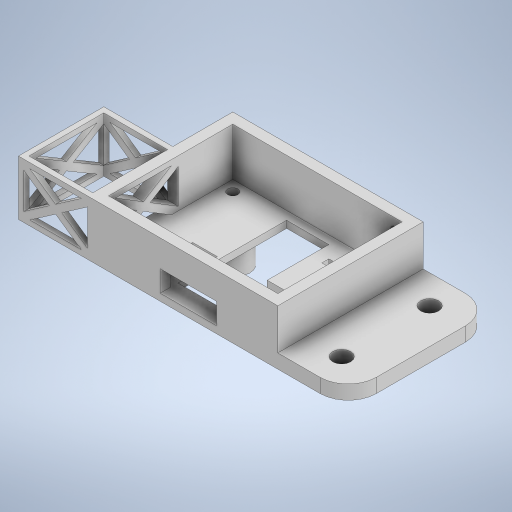
# Autodesk Inventor part: Thermostat_mount
Saved by Autodesk Inventor 2024 (Build 280153000, 153)
## iProperties
Created: 2024-10-23
Part Number: Thermostat_mount
Material: Generic
Document SubType Name: Modeling
Designer: Owner
Density: 1 g/cm^3
Appearance: Default
Author: Owner
Autodesk Inventor part; units mm, degrees
ref_plane "YZ Plane" through (0, 0, 0) normal (1, 0, 0) x (0, 1, 0)
ref_plane "XZ Plane" through (0, 0, 0) normal (0, 1, 0) x (-1, 0, 0)
ref_plane "XY Plane" through (0, 0, 0) normal (0, 0, 1) x (1, 0, 0)
sketch "Sketch1" plane through (0, 0, 0) normal (0, 1, 0) x (-1, 0, 0)
  line L0 (-30.0355, 21.9075) -> (30.0355, 21.9075)
  line L1 (30.0355, 21.9075) -> (30.0355, -21.9075)
  line L2 (30.0355, -21.9075) -> (-30.0355, -21.9075)
  line L3 (-30.0355, -21.9075) -> (-30.0355, 21.9075)
  line L4 (-30.0355, 21.9075) -> (30.0355, -21.9075) construction
  line L5 (30.0355, 21.9075) -> (-30.0355, -21.9075) construction
  line L6 (-30.5435, -22.4155) -> (30.5435, -22.4155)
  line L7 (30.5435, -22.4155) -> (30.5435, 22.4155)
  line L8 (30.5435, 22.4155) -> (-30.5435, 22.4155)
  line L9 (-30.5435, 22.4155) -> (-30.5435, -22.4155)
  line L10 (-28.3845, -20.2565) -> (28.3845, -20.2565)
  line L11 (28.3845, -20.2565) -> (28.3845, 20.2565)
  line L12 (28.3845, 20.2565) -> (-28.3845, 20.2565)
  line L13 (-28.3845, 20.2565) -> (-28.3845, -20.2565)
  line L14 (28.3845, -20.2565) -> (24.9555, -20.2565)
  line L15 (24.9555, -20.2565) -> (24.9555, -16.8275)
  line L16 (24.9555, -16.8275) -> (28.3845, -16.8275)
  line L17 (28.3845, -16.8275) -> (28.3845, -20.2565)
  line L18 (-28.3845, -20.2565) -> (-24.9555, -20.2565)
  line L19 (-24.9555, -20.2565) -> (-24.9555, -16.8275)
  line L20 (-24.9555, -16.8275) -> (-28.3845, -16.8275)
  line L21 (-28.3845, -16.8275) -> (-28.3845, -20.2565)
  line L22 (28.3845, 20.2565) -> (24.9555, 20.2565)
  line L23 (24.9555, 20.2565) -> (24.9555, 16.8275)
  line L24 (24.9555, 16.8275) -> (28.3845, 16.8275)
  line L25 (28.3845, 16.8275) -> (28.3845, 20.2565)
  line L26 (-28.3845, 20.2565) -> (-24.9555, 20.2565)
  line L27 (-24.9555, 20.2565) -> (-24.9555, 16.8275)
  line L28 (-24.9555, 16.8275) -> (-28.3845, 16.8275)
  line L29 (-28.3845, 16.8275) -> (-28.3845, 20.2565)
  circle A0 centre (26.67, -18.542) radius 1.7145
  circle A1 centre (-26.67, -18.542) radius 1.7145
  circle A2 centre (-26.67, 18.542) radius 1.7145
  circle A3 centre (26.67, 18.542) radius 1.7145
  circle A4 centre (26.67, -18.542) radius 1.8415
  circle A5 centre (-26.67, -18.542) radius 1.8415
  circle A6 centre (-26.67, 18.542) radius 1.8415
  circle A7 centre (26.67, 18.542) radius 1.8415
  line L30 (-28.3845, -20.2565) -> (-28.3845, -10.0965)
  line L31 (-30.0355, -21.9075) -> (-30.0355, -11.7475)
  line L32 (-30.0355, -11.7475) -> (-27.4955, -11.7475)
  line L33 (-27.4955, -11.7475) -> (-21.3995, -11.7475)
  line L34 (-21.3995, -11.7475) -> (-21.3995, -4.1275)
  line L35 (-21.3995, -4.1275) -> (-27.4955, -4.1275)
  line L36 (-27.4955, -4.1275) -> (-27.4955, -11.7475)
  line L37 (-30.0355, -21.9075) -> (-14.1605, -21.9075)
  line L38 (-14.1605, -21.9075) -> (-14.1605, -13.6525)
  line L39 (-16.7005, -14.9225) -> (-11.6205, -14.9225)
  line L40 (-11.6205, -14.9225) -> (-11.6205, -12.3825)
  line L41 (-11.6205, -12.3825) -> (-16.7005, -12.3825)
  line L42 (-16.7005, -12.3825) -> (-16.7005, -14.9225)
  line L43 (-16.7005, -14.9225) -> (-11.6205, -12.3825) construction
  line L44 (-11.6205, -14.9225) -> (-16.7005, -12.3825) construction
  line L45 (-30.0355, -21.9075) -> (-7.1755, -21.9075)
  line L46 (-7.1755, -21.9075) -> (-7.1755, -19.3675)
  line L47 (-7.1755, -19.3675) -> (8.0645, -19.3675)
  line L48 (8.0645, -19.3675) -> (8.0645, 2.2225)
  line L49 (8.0645, 2.2225) -> (-7.1755, 2.2225)
  line L50 (-7.1755, 2.2225) -> (-7.1755, -19.3675)
  line L51 (-30.0355, 21.9075) -> (-18.6055, 21.9075)
  line L52 (-18.6055, 21.9075) -> (-18.6055, 13.0175)
  line L53 (-18.6055, 13.0175) -> (8.0645, 13.0175)
  line L54 (8.0645, 13.0175) -> (8.0645, 2.8575)
  line L55 (8.0645, 2.8575) -> (-18.6055, 2.8575)
  line L56 (-18.6055, 2.8575) -> (-18.6055, 13.0175)
  line L57 (-30.0355, 21.9075) -> (-12.2555, 21.9075)
  line L58 (-12.2555, 21.9075) -> (-12.2555, 19.8755)
  line L59 (-12.2555, 19.8755) -> (8.0645, 19.8755)
  line L60 (8.0645, 19.8755) -> (8.0645, 16.0655)
  line L61 (8.0645, 16.0655) -> (-12.2555, 16.0655)
  line L62 (-12.2555, 16.0655) -> (-12.2555, 19.8755)
  line L63 (30.0355, 21.9075) -> (23.0505, 21.9075)
  line L64 (23.0505, 21.9075) -> (19.2405, 21.9075)
  line L65 (19.2405, 21.9075) -> (19.2405, 7.6835)
  line L66 (19.2405, 7.6835) -> (23.0505, 7.6835)
  line L67 (23.0505, 7.6835) -> (23.0505, 21.9075)
  line L68 (30.0355, 21.9075) -> (18.0975, 21.9075)
  line L69 (18.0975, 21.9075) -> (18.0975, 10.4775)
  line L70 (18.0975, 10.4775) -> (9.2075, 10.4775)
  line L71 (9.2075, 10.4775) -> (9.2075, 4.5085)
  line L72 (9.2075, 4.5085) -> (18.0975, 4.5085)
  line L73 (18.0975, 4.5085) -> (18.0975, 10.4775)
  point P0 (0, 0)
  point P1 (-28.3845, -19.214)
  point P2 (-28.3845, -18.542)
  point P3 (-26.67, -16.8275)
  point P4 (-27.342, -16.8275)
  point P5 (23.0505, 20.2565)
  point P6 (19.2405, 20.2565)
  dimension "d0" = 60.071
  dimension "d1" = 43.815
  dimension "d2" = 0.508
  dimension "d3" = 1.651
  dimension "d4" = 3.429
  dimension "d5" = 3.429
  dimension "d6" = 3.429
  dimension "d7" = 3.429
  dimension "d8" = 3.429
  dimension "d9" = 3.683
  dimension "d10" = 3.683
  dimension "d11" = 3.683
  dimension "d12" = 3.683
  dimension "d18" = 10.16
  dimension "d19" = 10.16
  dimension "d20" = 2.54
  dimension "d21" = 6.096
  dimension "d22" = 7.62
  dimension "d23" = 15.875
  dimension "d24" = 8.255
  dimension "d25" = 5.08
  dimension "d26" = 2.54
  dimension "d27" = 22.86
  dimension "d28" = 2.54
  dimension "d29" = 15.24
  dimension "d30" = 21.59
  dimension "d31" = 11.43
  dimension "d32" = 8.89
  dimension "d33" = 26.67
  dimension "d34" = 10.16
  dimension "d35" = 17.78
  dimension "d36" = 2.032
  dimension "d37" = 20.32
  dimension "d38" = 3.81
  dimension "d39" = 6.985
  dimension "d40" = 3.81
  dimension "d41" = 14.224
  dimension "d42" = 11.938
  dimension "d43" = 11.43
  dimension "d44" = 8.89
  dimension "d45" = 5.969
  constraints: 148 end point, 28 parallel, 20 perpendicular, 12 horizontal, 12 tangent, 11 point on line, 8 centre point, 4 coincident, 4 midpoint, 6 other
  measures "d0" distance of L1.end L2.end
  measures "d1" distance of L0.end L1.end
  measures "d2" distance between parallel lines of L2 L6
  measures "d3" distance between parallel lines of L2 L10
  measures "d4" distance of L15.end L16.end
  measures "d5" distance of L14.end L15.end
  measures "d6" distance of L20.end L19.end
  measures "d7" distance of L19.end L18.end
  measures "d8" distance of L23.end L22.end
  measures "d9" diameter of A4
  measures "d10" diameter of A5
  measures "d11" diameter of A6
  measures "d12" diameter of A7
  measures "d18" distance of L10.start L30.end
  measures "d19" distance of L2.end L31.end
  measures "d20" distance of L31.end L32.end
  measures "d21" distance of L35.end L34.end
  measures "d22" distance of L34.end L33.end
  measures "d23" distance of L2.end L37.end
  measures "d24" distance of L37.end L38.end
  measures "d25" distance of L41.end L40.end
  measures "d26" distance of L40.end L39.end
  measures "d27" distance of L2.end L45.end
  measures "d28" distance of L45.end L46.end
  measures "d29" distance of L49.end L48.end
  measures "d30" distance of L48.end L47.end
  measures "d31" distance of L0.start L51.end
  measures "d32" distance of L51.end L52.end
  measures "d33" distance of L54.end L55.end
  measures "d34" distance of L53.end L54.end
  measures "d35" distance of L0.start L57.end
  measures "d36" distance of L57.end L58.end
  measures "d37" distance of L60.end L61.end
  measures "d38" distance of L59.end L60.end
  measures "d39" distance of L0.end L63.end
  measures "d40" distance of L66.end L65.end
  measures "d41" distance of L65.end L64.end
  measures "d42" distance of L0.end L68.end
  measures "d43" distance of L68.end L69.end
  measures "d44" distance of L72.end L71.end
  measures "d45" distance of L71.end L70.end
extrude "Extrusion1" add sketch "Sketch1" along normal blind 2.54 contours L0 L52 L12 A6 L13 L32 L3 | L0 L58 L12 L52 | L32 L13 A5 L10 L38 L2 L3 | L0 L69 L12 L58 | L12 L65 L66 L67 L23 A7 L24 L11 L16 A4 L15 L10 L19 A5 L20 L13 L28 A6 L27 | L0 L65 L12 L69 | L27 A6 L12 | L38 L10 L46 L2 | L20 A5 L13 | L0 L67 L12 L65 | L46 L10 A4 L11 A7 L12 L67 L0 L1 L2 | L13 A6 L28 | A5 L20 A1 L13 | L13 A5 | A6 L13 L12 | L10 A5 L19 | A5 L10 L13 | L20 L19 A5 | L27 L28 A6 | L15 A4 L10 | L12 A7 L23 | A4 L11 L10 | L15 L16 A4 | L12 L11 A7 | A7 L24 L23 | A4 L16 L11 | L11 L24 A7 | L9 L8 L7 L6
sketch "Sketch2" plane through (0, 0, 0) normal (0, -1, 0) x (1, 0, 0)
  line L0 (-30.5435, 22.4155) -> (30.5435, 22.4155) projected
  line L1 (-30.5435, -22.4155) -> (30.5435, -22.4155)
  line L2 (30.5435, -22.4155) -> (30.5435, 22.4155)
  line L3 (30.5435, 22.4155) -> (-30.5435, 22.4155)
  line L4 (-30.5435, 22.4155) -> (-30.5435, -22.4155)
  line L5 (-30.5435, -22.4155) -> (30.5435, 22.4155) construction
  line L6 (30.5435, -22.4155) -> (-30.5435, 22.4155) construction
  line L7 (-34.3535, -26.2255) -> (34.3535, -26.2255)
  line L8 (34.3535, -26.2255) -> (34.3535, 26.2255)
  line L9 (34.3535, 26.2255) -> (-34.3535, 26.2255)
  line L10 (-34.3535, 26.2255) -> (-34.3535, -26.2255)
  line L11 (-30.5435, 22.4155) -> (-34.3535, 22.4155)
  line L12 (-34.3535, 22.4155) -> (34.3535, 22.4155)
  line L13 (-34.3535, -22.4155) -> (34.3535, -22.4155)
  point P0 (0, 0)
  dimension "d15" = 3.81
  constraints: 26 end point, 7 point on line, 4 parallel, 3 perpendicular, 2 midpoint, 1 horizontal, 3 other
  measures "d15" distance between parallel lines of L4 L10
extrude "Extrusion2" add sketch "Sketch2" against normal blind 19.812 contours L11 L10 L9 L8 L12 L0 | L4 L13 L10 L11 | L12 L8 L13 L2 | L1 L13 L8 L7 L10
sketch "Sketch3" plane through (-34.3535, 0, 26.2255) normal (0, 0, 1) x (1, 0, 0)
  line L0 (3.81, 2.54) -> (64.897, 2.54) projected
  line L1 (64.897, 2.54) -> (68.707, 2.54)
  line L2 (68.707, 0) -> (68.707, 19.812) projected
  line L3 (64.897, 2.54) -> (64.897, 0)
  line L4 (68.707, 2.54) -> (46.609, 2.54)
  line L5 (46.609, 2.54) -> (26.289, 2.54)
  line L6 (26.289, 2.54) -> (26.289, 10.16)
  line L7 (26.289, 10.16) -> (46.609, 10.16)
  line L8 (46.609, 10.16) -> (46.609, 2.54)
  point P0 (34.3535, 0)
  point P1 (26.289, 2.54)
  dimension "d46" = 22.098
  dimension "d47" = 20.32
  dimension "d48" = 7.62
  constraints: 14 end point, 2 horizontal, 2 parallel, 2 point on line, 1 perpendicular, 1 vertical
  measures "d46" distance of L1.end L4.end
  measures "d47" distance of L6.end L7.end
  measures "d48" distance of L5.end L6.end
extrude "Extrusion3" cut sketch "Sketch3" against normal blind 3.81
sketch "Sketch4" plane through (34.3535, 0, 26.2255) normal (1, 0, 0) x (0, 0, -1)
  line L0 (52.451, 0) -> (0, 0) projected
  line L1 (0, 10.16) -> (0, 2.54) projected
  line L2 (52.451, 0) -> (0, 0)
  line L3 (0, 0) -> (0, 5.08)
  line L4 (0, 5.08) -> (52.451, 5.08)
  line L5 (52.451, 5.08) -> (52.451, 0)
  point P0 (26.2255, 0)
  dimension "d51" = 5.08
  constraints: 8 end point, 2 parallel, 1 horizontal, 1 perpendicular, 1 point on line
  measures "d51" distance of L2.end L3.end
extrude "Extrusion4" add sketch "Sketch4" along normal blind 25.4
sketch "Sketch5" plane through (34.3535, 5.08, 26.2255) normal (0, 1, 0) x (1, 0, 0)
  line L0 (-68.707, 52.451) -> (25.4, 52.451) projected
  line L1 (0, 0) -> (0, 52.451) projected
  line L2 (25.4, 52.451) -> (0, 52.451)
  line L3 (0, 52.451) -> (0, 0)
  line L4 (0, 0) -> (25.4, 0)
  line L5 (25.4, 0) -> (25.4, 52.451)
  line L6 (12.7, 52.451) -> (12.7, 0)
  line L7 (25.4, 26.2255) -> (0, 26.2255)
  line L8 (0, 10.3505) -> (25.4, 10.3505)
  line L9 (25.4, 10.3505) -> (25.4, 42.1005)
  line L10 (25.4, 42.1005) -> (0, 42.1005)
  line L11 (0, 42.1005) -> (0, 10.3505)
  line L12 (0, 10.3505) -> (25.4, 42.1005) construction
  line L13 (25.4, 10.3505) -> (0, 42.1005) construction
  circle A0 centre (12.7, 42.1005) radius 3.2385
  circle A1 centre (12.7, 10.3505) radius 3.2385
  point P0 (-34.3535, 26.2255)
  point P1 (12.7, 26.2255)
  dimension "d54" = 25.4
  dimension "d55" = 31.75
  dimension "d56" = 6.477
  dimension "d57" = 6.477
  constraints: 24 end point, 9 midpoint, 4 parallel, 2 centre point, 2 horizontal, 2 perpendicular
  measures "d54" distance of L10.end L9.end
  measures "d55" distance of L9.end L8.end
  measures "d56" diameter of A0
  measures "d57" diameter of A1
extrude "Extrusion5" cut sketch "Sketch5" against normal blind 25.4 contours A0 L10 L6 | L6 L10 A0 | L10 L6 A0 | L10 A0 L6 | A1 L6 L8 | L8 L6 A1 | A1 L8 L6 | L8 A1 L6
fillet "Fillet1" radius 10.16 2 edges at (59.7535, 2.54, -26.2255) (59.7535, 2.54, 26.2255)
sketch "Sketch6" plane through (0, 0, 0) normal (0, -1, 0) x (1, 0, 0)
  circle A0 centre (-26.67, -18.542) radius 1.8415 projected
  line L0 (-24.8285, -18.542) -> (-5.6313, -18.542)
  line L1 (-5.6313, -18.542) -> (-5.6313, 2.1308)
  line L2 (-5.6313, 2.1308) -> (-24.8285, 2.1308)
  line L3 (-24.8285, 2.1308) -> (-24.8285, -18.542)
  line L4 (-5.6313, -8.2056) -> (-24.8285, -8.2056)
  line L5 (-15.2299, -18.542) -> (-15.2299, 2.1308)
  circle A1 centre (-15.2299, -8.2056) radius 5.08
  point P0 (0, 0)
  dimension "d61" = 10.16
  constraints: 12 end point, 5 midpoint, 2 parallel, 1 centre point, 1 horizontal, 1 horizontal alignment, 1 perpendicular, 1 other
  measures "d61" diameter of A1
extrude "Extrusion6" add sketch "Sketch6" along normal blind 9.398 contours A1 L4 L5 | L5 L4 A1 | A1 L5 L4 | L5 A1 L4
sketch "Sketch7" plane through (0, 0, 0) normal (0, -1, 0) x (1, 0, 0)
  line L0 (-8.0645, 2.2225) -> (-8.0645, -19.3675) projected
  line L1 (-8.0645, 2.2225) -> (-8.0645, 2.8575)
  line L2 (-8.0645, 2.8575) -> (18.6055, 2.8575) projected
  line L3 (7.1755, -19.3675) -> (7.1755, 2.2225) projected
  line L4 (7.1755, 2.2225) -> (-8.0645, 2.2225)
  line L5 (-8.0645, 2.2225) -> (-8.0645, 2.8575)
  line L6 (-8.0645, 2.8575) -> (7.1755, 2.8575)
  line L7 (7.1755, 2.8575) -> (7.1755, 2.2225)
  point P0 (0, 0)
  point P1 (7.1755, 2.8575)
  constraints: 10 end point, 2 parallel, 1 horizontal, 1 perpendicular, 1 point on line, 1 vertical
extrude "Extrusion7" cut sketch "Sketch7" against normal blind 9.398
sketch "Sketch8" plane through (34.3535, 19.812, -26.2255) normal (0, 0, -1) x (-1, 0, 0)
  line L0 (22.098, -17.272) -> (3.81, -17.272) projected
  line L1 (3.81, 0) -> (64.897, 0) projected
  line L2 (3.81, -17.272) -> (3.81, 0)
  line L3 (59.182, -17.272) -> (62.865, -17.272) projected
  line L4 (3.81, -17.272) -> (62.865, -17.272)
  circle A0 centre (5.969, -4.6996) radius 2.159
  point P0 (34.3535, -19.812)
  dimension "d66" = 4.318
  constraints: 4 end point, 1 centre point, 1 horizontal, 1 perpendicular, 1 tangent
  measures "d66" diameter of A0
extrude "Extrusion8" cut sketch "Sketch8" against normal blind 25.4
sketch "Sketch9" plane through (0, 0, 0) normal (0, -1, 0) x (1, 0, 0)
  line L0 (-34.3535, 26.2255) -> (-34.3535, 24.3205)
  line L1 (-34.3535, 26.2255) -> (-34.3535, -26.2255) projected
  line L2 (-34.3535, 24.3205) -> (-57.3535, 24.3205)
  line L3 (-57.3535, 24.3205) -> (-57.3535, -2.6795)
  line L4 (-57.3535, -2.6795) -> (-34.3535, -2.6795)
  line L5 (-34.3535, -2.6795) -> (-34.3535, 24.3205)
  line L6 (-59.2585, -4.5845) -> (-59.2585, 26.2255)
  line L7 (-59.2585, 26.2255) -> (-32.4485, 26.2255)
  line L8 (-32.4485, 26.2255) -> (-32.4485, -4.5845)
  line L9 (-32.4485, -4.5845) -> (-59.2585, -4.5845)
  line L10 (-34.3535, 26.2255) -> (-34.3535, -4.5845)
  point P0 (0, 0)
  dimension "d69" = 1.905
  dimension "d70" = 23
  dimension "d71" = 27
  dimension "d72" = 1.905
  constraints: 20 end point, 4 parallel, 3 point on line, 2 perpendicular, 1 horizontal, 3 other
  measures "d69" distance of L0.start L0.end
  measures "d70" distance of L4.end L3.end
  measures "d71" distance of L3.end L2.end
  measures "d72" distance between parallel lines of L3 L6
extrude "Extrusion9" add sketch "Sketch9" against normal up to surface (19.812 mm away) contours L0 L2 L3 L4 L1 L9 L6 L7
sketch "Sketch10" plane through (-34.3535, 0, -2.6795) normal (-1, 0, 0) x (0, 0, 1)
  line L0 (0, 19.812) -> (27, 19.812) projected
  line L1 (0, 19.812) -> (0, 0) projected
  line L2 (27, 19.812) -> (0, 19.812)
  line L3 (0, 19.812) -> (0, 17.907)
  line L4 (0, 17.907) -> (27, 17.907)
  line L5 (27, 17.907) -> (27, 19.812)
  point P0 (2.6795, 0)
  dimension "d75" = 1.905
  constraints: 8 end point, 2 parallel, 1 horizontal, 1 perpendicular, 1 point on line
  measures "d75" distance of L3.end L2.end
extrude "Extrusion10" add sketch "Sketch10" along normal up to surface (23 mm away)
sketch "Sketch11" plane through (34.3535, 5.08, 26.2255) normal (0, 0, 1) x (1, 0, 0)
  line L0 (-91.707, 12.827) -> (-68.707, 12.827) projected
  line L1 (-91.707, -5.08) -> (-91.707, 12.827) projected
  line L2 (-68.707, 12.827) -> (-91.707, 12.827)
  line L3 (-91.707, 12.827) -> (-91.707, -3.175)
  line L4 (-91.707, -3.175) -> (-68.707, -3.175)
  line L5 (-68.707, -3.175) -> (-68.707, 12.827)
  line L6 (-91.707, 12.827) -> (-68.707, -3.175)
  line L7 (-91.707, -3.175) -> (-68.707, 12.827)
  line L8 (-90.9817, 13.8695) -> (-67.9817, -2.1325)
  line L9 (-92.4323, 11.7845) -> (-69.4323, -4.2175)
  line L10 (-92.4323, -2.1325) -> (-69.4323, 13.8695)
  line L11 (-90.9817, -4.2175) -> (-67.9817, 11.7845)
  point P0 (-34.3535, -5.08)
  point P1 (-80.207, 3.2789)
  point P2 (-89.4833, -3.175)
  point P3 (-70.9307, -3.175)
  point P4 (-68.707, 11.2799)
  point P5 (-77.9833, 4.826)
  point P6 (-68.707, -1.6279)
  point P7 (-91.707, -1.6279)
  point P8 (-82.4307, 4.826)
  point P9 (-91.707, 11.2799)
  point P10 (-80.207, 6.3731)
  point P11 (-70.9307, 12.827)
  point P12 (-89.4833, 12.827)
  dimension "d78" = 16.002
  dimension "d79" = 1.27
  dimension "d80" = 1.27
  dimension "d81" = 1.27
  dimension "d82" = 1.27
  constraints: 20 end point, 6 parallel, 1 horizontal, 1 perpendicular, 1 point on line
  measures "d78" distance of L3.end L2.end
  measures "d79" distance between parallel lines of L6 L8
  measures "d80" distance between parallel lines of L6 L9
  measures "d81" distance between parallel lines of L7 L10
  measures "d82" distance between parallel lines of L7 L11
extrude "Extrusion11" cut sketch "Sketch11" against normal blind 50.8 contours L0 L10 L8 | L9 L10 L1 | L5 L8 L11 | L11 L9 L4
sketch "Sketch12" plane through (-59.2585, 0, -4.5845) normal (-1, 0, 0) x (0, 0, 1)
  line L0 (1.905, 17.907) -> (28.905, 17.907) projected
  line L1 (1.905, 17.907) -> (28.9052, 17.907)
  line L2 (28.9052, 17.907) -> (28.9052, 1.905)
  line L3 (28.9052, 1.905) -> (1.905, 1.905)
  line L4 (1.905, 1.905) -> (1.905, 17.907)
  line L5 (1.905, 17.907) -> (28.9052, 1.905)
  line L6 (1.905, 1.905) -> (28.9052, 17.907)
  line L7 (1.2575, 2.9975) -> (28.2577, 18.9995)
  line L8 (2.5525, 0.8125) -> (29.5527, 16.8145)
  line L9 (2.5525, 18.9995) -> (29.5527, 2.9975)
  line L10 (1.2575, 16.8145) -> (28.2577, 0.8125)
  point P0 (4.5845, 0)
  point P1 (26.4143, 1.905)
  point P2 (15.4051, 8.4297)
  point P3 (4.3959, 1.905)
  point P4 (17.896, 9.906)
  point P5 (28.9052, 3.3813)
  point P6 (28.9052, 16.4307)
  point P7 (12.9142, 9.906)
  point P8 (1.905, 16.4307)
  point P9 (1.905, 3.3813)
  point P10 (4.3959, 17.907)
  point P11 (15.4051, 11.3823)
  point P12 (26.4143, 17.907)
  dimension "d85" = 27.0002
  dimension "d86" = 16.002
  dimension "d87" = 1.27
  dimension "d88" = 1.27
  dimension "d89" = 1.27
  dimension "d90" = 1.27
  constraints: 20 end point, 6 parallel, 1 horizontal, 1 perpendicular
  measures "d85" distance of L2.end L3.end
  measures "d86" distance of L1.end L2.end
  measures "d87" distance between parallel lines of L6 L7
  measures "d88" distance between parallel lines of L6 L8
  measures "d89" distance between parallel lines of L5 L9
  measures "d90" distance between parallel lines of L5 L10
extrude "Extrusion12" cut sketch "Sketch12" against normal blind 2.54 contours L0 L7 L9 | L10 L7 L4 | L2 L9 L8 | L8 L10 L3
sketch "Sketch13" plane through (-30.5435, 2.54, -22.4155) normal (1, 0, 0) x (0, 0, -1)
  line L0 (-44.831, 17.272) -> (-44.831, 15.367)
  line L1 (-19.736, 15.367) -> (-19.736, 13.8199) projected
  line L2 (-44.831, 15.367) -> (-19.736, 15.367)
  line L3 (-19.736, 15.367) -> (-19.736, 0)
  line L4 (0, 0) -> (-44.831, 0) projected
  line L5 (-19.736, 0) -> (-44.831, 0)
  line L6 (-44.831, 0) -> (-44.831, 15.367)
  line L7 (-19.736, 0) -> (-44.831, 15.367)
  line L8 (-44.831, 0) -> (-19.736, 15.367)
  line L9 (-20.3992, -1.0831) -> (-45.4942, 14.2839)
  line L10 (-19.0728, 1.0831) -> (-44.1678, 16.4501)
  line L11 (-45.4942, 1.0831) -> (-20.3992, 16.4501)
  line L12 (-44.1678, -1.0831) -> (-19.0728, 14.2839)
  point P0 (-22.4155, -2.54)
  point P1 (-19.736, 13.8778)
  point P2 (-29.8516, 7.6835)
  point P3 (-19.736, 1.4892)
  point P4 (-32.2835, 9.1727)
  point P5 (-22.1679, 15.367)
  point P6 (-42.3991, 15.367)
  point P7 (-32.2835, 6.1943)
  point P8 (-42.3991, 0)
  point P9 (-22.1679, 0)
  point P10 (-44.831, 1.4892)
  point P11 (-34.7154, 7.6835)
  point P12 (-44.831, 13.8778)
  dimension "d93" = 1.905
  dimension "d94" = 1.27
  dimension "d95" = 1.27
  dimension "d96" = 1.27
  dimension "d97" = 1.27
  constraints: 22 end point, 4 parallel, 2 vertical, 1 collinear, 1 point on line
  measures "d93" distance of L0.start L0.end
  measures "d94" distance between parallel lines of L7 L9
  measures "d95" distance between parallel lines of L7 L10
  measures "d96" distance between parallel lines of L8 L11
  measures "d97" distance between parallel lines of L8 L12
extrude "Extrusion13" cut sketch "Sketch13" against normal blind 5.08 contours L1 L3 L10 L12 | L11 L10 L2 | L9 L4 L12 | L9 L11 L6
sketch "Sketch14" plane through (0, 19.812, 0) normal (0, 1, 0) x (1, 0, 0)
  line L0 (-34.3535, 2.6795) -> (-34.3535, 4.5845) projected
  line L1 (-57.3535, -21.8298) -> (-57.3535, -24.3205) projected
  line L2 (-34.3535, 2.6795) -> (-57.3535, 2.6795)
  line L3 (-57.3535, 2.6795) -> (-57.3535, -24.3205)
  line L4 (-57.3535, -24.3205) -> (-34.3535, -24.3205)
  line L5 (-34.3535, -24.3205) -> (-34.3535, 2.6795)
  line L6 (-57.3535, 2.6795) -> (-34.3535, -24.3205)
  line L7 (-34.3535, -24.3205) -> (-34.3535, 2.6795) projected
  line L8 (-57.3535, -26.2255) -> (-57.3535, -24.3207) projected
  line L9 (-34.3535, 2.6795) -> (-57.3535, -24.3207)
  line L10 (-56.3867, 3.5031) -> (-33.3867, -23.4969)
  line L11 (-58.3203, 1.8559) -> (-35.3203, -25.1441)
  line L12 (-35.3203, 3.503) -> (-58.6235, -23.8531)
  line L13 (-58.6235, -23.8531) -> (-58.6235, -26.2255)
  line L14 (-33.3867, 1.856) -> (-56.0835, -24.7883)
  line L15 (-56.0835, -24.7883) -> (-56.0835, -26.2255)
  line L16 (-50.9335, -16.7841) -> (-40.7735, -16.7841)
  line L17 (-40.7735, -16.7841) -> (-40.7735, -4.8571)
  line L18 (-40.7735, -4.8571) -> (-50.9335, -4.8571)
  line L19 (-50.9335, -4.8571) -> (-50.9335, -16.7841)
  line L20 (-50.9335, -16.7841) -> (-40.7735, -4.8571) construction
  line L21 (-40.7735, -16.7841) -> (-50.9335, -4.8571) construction
  point P0 (0, 0)
  point P1 (-45.8535, -10.8206)
  point P2 (-42.4417, -16.7841)
  point P3 (-49.2652, -16.7841)
  point P4 (-55.685, -24.3205)
  point P5 (-36.0218, -24.3205)
  point P6 (-40.7735, -6.8156)
  point P7 (-40.7735, -14.8255)
  point P8 (-34.3535, -22.362)
  point P9 (-34.3535, 0.721)
  point P10 (-50.9335, -14.8256)
  point P11 (-50.9335, -6.8155)
  point P12 (-57.3535, 0.721)
  point P13 (-57.3535, -22.3622)
  point P14 (-49.2651, -4.8571)
  point P15 (-42.4418, -4.8571)
  point P16 (-36.0218, 2.6795)
  point P17 (-55.6852, 2.6795)
  dimension "d100" = 1.27
  dimension "d101" = 1.27
  dimension "d102" = 1.27
  dimension "d103" = 1.27
  dimension "d104" = 10.16
  constraints: 36 end point, 6 parallel, 3 midpoint, 2 horizontal, 2 perpendicular, 1 point on line, 2 other
  measures "d100" distance between parallel lines of L6 L10
  measures "d101" distance between parallel lines of L6 L11
  measures "d102" distance between parallel lines of L9 L12
  measures "d103" distance between parallel lines of L9 L14
  measures "d104" distance of L18.end L17.end
extrude "Extrusion14" cut sketch "Sketch14" against normal blind 5.08 contours L3 L11 L19 L12 L1 | L14 L16 L11 L4 | L2 L12 L18 L10 | L10 L17 L14 L5
sketch "Sketch15" plane through (0, 19.812, 0) normal (0, 1, 0) x (1, 0, 0)
  line L0 (-55.6852, 2.6795) -> (-57.3535, 2.6795) projected
  line L1 (-57.3535, 2.6795) -> (-34.3535, 2.6795)
  line L2 (-34.3535, 2.6795) -> (-34.3535, -24.3205)
  line L3 (-34.3535, -24.3205) -> (-57.3535, -24.3205)
  line L4 (-57.3535, -24.3205) -> (-57.3535, 2.6795)
  point P0 (0, 0)
  constraints: 8 end point, 2 parallel, 1 horizontal, 1 perpendicular
extrude "Extrusion15" cut sketch "Sketch15" against normal blind 25.4
body "Solid1"
